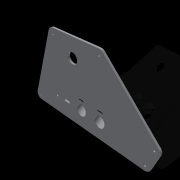
# Autodesk Inventor part: switchback-primary-cover
Saved by Autodesk Inventor 2020 (Build 240168000, 168)
## iProperties
Created: 2020-01-08
Part Number: switchback-primary-cover
Material: Generic
Document SubType Name: Modeling
Designer: valer
Density: 1 g/cm^3
Appearance: Default
Author: valer
Autodesk Inventor part; units mm, degrees
ref_plane "XZ Plane" through (0, 0, 0) normal (0, 1, 0) x (-1, 0, 0)
ref_plane "XY Plane" through (0, 0, 0) normal (0, 0, 1) x (1, 0, 0)
sketch "Profile" plane through (0, 0, 0) normal (0, 0, 1) x (1, 0, 0)
  circle A0 centre (1234.4703, 243.0527) radius 1.27
  circle A1 centre (1077.082, 219.7111) radius 1.27
  circle A2 centre (1109.7778, 307.7683) radius 1.27
  circle A3 centre (1169.7547, 307.7683) radius 1.27
  circle A4 centre (1228.2159, 219.7111) radius 1.27
  line L0 (1232.1045, 221.9562) -> (1229.0377, 222.7779)
  arc A5 (1229.0377, 222.7779) -> (1225.0409, 219.7111) centre (1228.2159, 219.7111) ccw
  line L1 (1225.0409, 219.7111) -> (1225.0409, 216.5361)
  line L2 (1080.257, 216.5361) -> (1225.0409, 216.5361)
  line L3 (1080.257, 216.5361) -> (1080.257, 219.7111)
  arc A6 (1080.257, 219.7111) -> (1078.1871, 222.6876) centre (1077.082, 219.7111) ccw
  line L4 (1078.1871, 222.6876) -> (1075.2107, 223.7927)
  line L5 (1106.8013, 308.8734) -> (1075.2107, 223.7927)
  arc A7 (1106.8013, 308.8734) -> (1112.9528, 307.7683) centre (1109.7778, 307.7683) ccw
  line L6 (1112.9528, 307.7683) -> (1112.9528, 310.9433)
  line L7 (1166.5797, 310.9433) -> (1112.9528, 310.9433)
  line L8 (1166.5797, 310.9433) -> (1166.5797, 307.7683)
  arc A8 (1166.5797, 307.7683) -> (1171.9998, 305.5232) centre (1169.7547, 307.7683) ccw
  line L9 (1171.9998, 305.5232) -> (1174.2448, 307.7683)
  line L10 (1234.4703, 247.5428) -> (1174.2448, 307.7683)
  line L11 (1234.4703, 247.5428) -> (1232.2252, 245.2978)
  arc A9 (1232.2252, 245.2978) -> (1233.6485, 239.9859) centre (1234.4703, 243.0527) ccw
  line L12 (1233.6485, 239.9859) -> (1236.7153, 239.1642)
  line L13 (1232.1045, 221.9562) -> (1236.7153, 239.1642)
  arc A10 (1109.7778, 314.1183) -> (1103.8249, 309.9786) centre (1109.7778, 307.7683) ccw
  line L14 (1071.1291, 221.9214) -> (1103.8249, 309.9786)
  arc A11 (1071.1291, 221.9214) -> (1077.082, 213.3611) centre (1077.082, 219.7111) ccw
  line L15 (1228.2159, 213.3611) -> (1077.082, 213.3611)
  arc A12 (1228.2159, 213.3611) -> (1234.3495, 218.0676) centre (1228.2159, 219.7111) ccw
  line L16 (1240.6039, 241.4092) -> (1234.3495, 218.0676)
  arc A13 (1240.6039, 241.4092) -> (1238.9604, 247.5428) centre (1234.4703, 243.0527) ccw
  line L17 (1174.2448, 312.2584) -> (1238.9604, 247.5428)
  arc A14 (1174.2448, 312.2584) -> (1169.7547, 314.1183) centre (1169.7547, 307.7683) ccw
  line L18 (1109.7778, 314.1183) -> (1169.7547, 314.1183)
  ellipse E0 centre (1136.6676, 291.8933) end of major axis (1136.6676, 298.2433) minor radius 6.3491
  circle A15 centre (1200.6281, 228.8981) radius 3.175 construction
  circle A16 centre (1175.2281, 228.8981) radius 3.175 construction
  circle A17 centre (1156.1781, 228.8981) radius 1.27 construction
  line L19 (1149.8281, 227.6281) -> (1156.1781, 227.6281) construction
  line L20 (1156.1781, 230.1681) -> (1149.8281, 230.1681) construction
  circle A18 centre (1149.8281, 228.8981) radius 1.27 construction
  circle A19 centre (1137.1281, 228.8981) radius 1.5875 construction
  point P0 (0, 0)
  constraints: 42 end point, 20 centre point, 20 point on circle, 2 other
extrude "ProfileFeature" add sketch "Profile" along normal blind 2.54 contours L0 A5 L1 L2 L3 A6 L4 L5 A7 L6 L7 L8 A8 L9 L10 L11 A9 L12 L13 | L18 A14 L17 A13 L16 A12 L15 A11 L14 A10
ref_plane "RouterPlaneFeature" through (1071.1291, 221.9214, 2.54) normal (1, 0, 0) x (0, 1, 0)
sketch "Sketch7" plane through (1071.1291, 221.9214, 2.54) normal (1, 0, 0) x (0, 1, 0)
  line L0 (0, 0) -> (-8.5603, 0) projected
  line L1 (88.0571, 0) -> (0, 0) projected
  line L2 (-8.5603, 0) -> (9.817, 23.5219)
  line L3 (9.817, 23.5219) -> (46.0375, 0)
  line L4 (0, 0) -> (-36.5125, 0)
  point P0 (-221.9214, -2.54)
  dimension "d48" = 52
  dimension "d49" = 33
  constraints: 6 end point, 2 point on line, 1 horizontal
  measures "d48" angle of L1 L2
  measures "d49" angle of L1 L3
extrude "RouterSideFeature" add sketch "Sketch7" along normal blind 127 separate body
extrude "RouterFeature" cut sketch "Profile" along normal blind 127 contours L0 A5 L1 L2 L3 A6 L4 L5 A7 L6 L7 L8 A8 L9 L10 L11 A9 L12 L13 keep common part bodies 2
combine bodies "RouterCombineFeature" operation type add bodies to combine 2 1
sketch "Panel" plane through (1078.1609, 231.7384, 26.0619) normal (0, 0.544639, 0.8386706) x (1, 0, 0)
  circle A0 centre (31.0681, 17.78) radius 1.5875
  circle A1 centre (43.7681, 17.78) radius 1.27
  line L0 (50.1181, 19.05) -> (43.7681, 19.05)
  line L1 (43.7681, 16.51) -> (50.1181, 16.51)
  circle A2 centre (50.1181, 17.78) radius 1.27
  circle A3 centre (69.1681, 17.78) radius 6.35
  circle A4 centre (94.5681, 17.78) radius 6.35
  line L2 (0, 0) -> (13.4487, 43.188) construction
  line L3 (0, 0) -> (119.9681, 0) construction
  line L4 (119.9681, 43.188) -> (119.9681, 0) construction
  line L5 (13.4487, 43.188) -> (119.9681, 43.188) construction
  line L6 (119.9681, 43.188) -> (119.9681, 0) construction
  line L7 (119.9681, 17.78) -> (5.5367, 17.78) construction
  line L8 (0, 0) -> (13.4487, 43.188) construction
  line L9 (13.4487, 43.188) -> (119.9681, 43.188) projected
  line L10 (119.9681, 0.0612) -> (119.9681, 43.188) projected
  point P0 (-1078.1609, -180.1579)
  dimension "d54" = 25.4
  dimension "d55" = 19.05
  dimension "d56" = 12.7
  dimension "d57" = 6.35
  dimension "d58" = 12.7
  dimension "d59" = 2.54
  dimension "d60" = 3.175
  dimension "d61" = 25.4
  dimension "d62" = 17.78
  constraints: 7 point on line, 6 end point, 5 centre point, 4 point on circle, 4 tangent, 2 equal radius, 1 parallel
  measures "d54" distance of A4.centre A3.centre
  measures "d55" distance of A3.centre A2.centre
  measures "d56" distance of A1.centre A0.centre
  measures "d57" distance of L0.start L0.end
  measures "d58" diameter of A4
  measures "d59" diameter of A2
  measures "d60" diameter of A0
  measures "d61" distance from line of L4 A4.centre
  measures "d62" distance between parallel lines of L3 L7
extrude "PanelFeature" cut sketch "Panel" against normal through all bodies 2
sketch "Countersinks" plane through (1078.1609, 231.7384, 26.0619) normal (0, 0.544639, 0.8386706) x (1, 0, 0)
  circle A0 centre (69.1681, 17.78) radius 6.35 projected
  arc A1 (50.1181, 16.51) -> (50.1181, 19.05) centre (50.1181, 17.78) ccw projected
  line L0 (50.1181, 16.51) -> (43.7681, 16.51) projected
  arc A2 (43.7681, 19.05) -> (43.7681, 16.51) centre (43.7681, 17.78) ccw projected
  line L1 (43.7681, 19.05) -> (50.1181, 19.05) projected
  circle A3 centre (94.5681, 17.78) radius 6.35 projected
  circle A4 centre (31.0681, 17.78) radius 1.5875 projected
  line L2 (0, 0) -> (13.4487, 43.188) projected
  line L3 (0, 0) -> (119.9681, 0) projected
  line L4 (119.9681, 43.188) -> (119.9681, 0) projected
  line L5 (13.4487, 43.188) -> (119.9681, 43.188) projected
  arc A5 (50.1181, 14.605) -> (50.1181, 20.955) centre (50.1181, 17.78) ccw
  line L6 (50.1181, 14.605) -> (43.7681, 14.605)
  arc A6 (43.7681, 20.955) -> (43.7681, 14.605) centre (43.7681, 17.78) ccw
  line L7 (43.7681, 20.955) -> (50.1181, 20.955)
  circle A7 centre (31.0681, 17.78) radius 4.2333
  circle A8 centre (69.1681, 17.78) radius 11.43
  circle A9 centre (94.5681, 17.78) radius 11.43
  point P0 (-1078.1609, -180.1579)
  dimension "d66" = 22.86
  dimension "d67" = 8.4667
  dimension "d68" = 1.905
  constraints: 5 centre point, 4 end point, 4 point on circle, 1 coincident, 1 equal radius, 3 other
  measures "d66" diameter of A8
  measures "d67" diameter of A7
  measures "d68" distance between parallel lines of L1 L7
extrude "CountersinksFeature" cut sketch "Countersinks" against normal blind 12.7 contours L6 A6 L7 A5 | A7 | A8 | A9 bodies 2
split "RouterTrimFeature" plane through (1077.082, 213.3611, 7.62) removes the side toward (0, 0, 1) bodies 2
ref_plane "RouterTrimPlane" through (1077.082, 213.3611, 7.62) normal (0, 0, -1) x (-1, 0, 0)
ref_plane "FlipPlane" through (1077.082, 213.3611, 2.54) normal (0, 0, 1) x (1, 0, 0)
mirror "FlipFeature" about plane through (1077.082, 213.3611, 2.54) normal (0, 0, 1) remove original yes bodies 2
body "Solid2"
